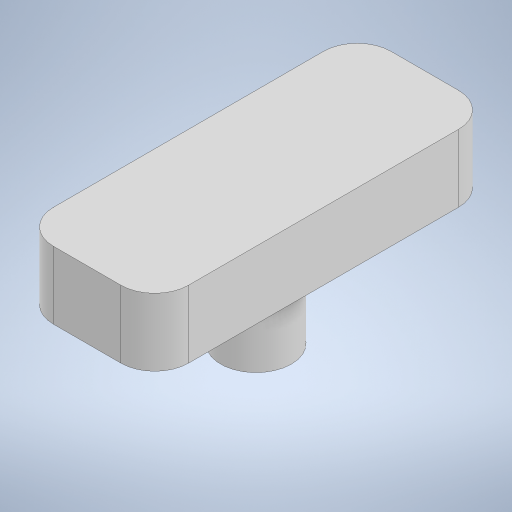
# Autodesk Inventor part: flipper_robot_v1_flipper_adapter
Saved by Autodesk Inventor 2023.1 (Build 271208000, 208)
## iProperties
Created: 2025-10-17
Part Number: flipper_robot_v1_flipper_adapter
Material: Generic
Document SubType Name: Modeling
Designer: Lars
Density: 1 g/cm^3
Appearance: Default
Author: Lars
Autodesk Inventor part; units mm, degrees
ref_plane "YZ Plane" through (0, 0, 0) normal (1, 0, 0) x (0, 1, 0)
ref_plane "XZ Plane" through (0, 0, 0) normal (0, 1, 0) x (-1, 0, 0)
ref_plane "XY Plane" through (0, 0, 0) normal (0, 0, 1) x (1, 0, 0)
sketch "Sketch1" plane through (0, 0, 0) normal (0, 1, 0) x (-1, 0, 0)
  line L0 (0.9994, -10) -> (3.0006, -10)
  ellipse E0 centre (2.9994, -8.9994) end of major axis (3.7074, -9.7074) minor radius 1 (3.0006, -10) -> (4, -9.0006) ccw
  line L1 (4, -9.0006) -> (4, -0.9994)
  ellipse E1 centre (2.9994, -1.0006) end of major axis (3.7074, -0.2926) minor radius 1 (4, -0.9994) -> (3.0006, 0) ccw
  line L2 (3.0006, 0) -> (0.9994, 0)
  ellipse E2 centre (1.0006, -1.0006) end of major axis (1.7086, -1.7086) minor radius 1 (0.9994, 0) -> (0, -0.9994) ccw
  line L3 (0, -0.9994) -> (0, -9.0006)
  ellipse E3 centre (1.0006, -8.9994) end of major axis (1.7086, -8.2914) minor radius 1 (0, -9.0006) -> (0.9994, -10) ccw
  circle A0 centre (2, -5) radius 1.75
  circle A1 centre (2, -5) radius 1.25
  line L4 (0, 0) -> (4, 0)
  line L5 (4, 0) -> (4, -10)
  line L6 (4, -10) -> (0, -10)
  line L7 (0, -10) -> (0, 0)
  circle A2 centre (2, -5) radius 1.05
  point P0 (0, -5)
  dimension "d3" = 1
  dimension "d7" = 1.0013
  dimension "d0" = 2.5
  dimension "d1" = 4
  dimension "d2" = 10
  dimension "d4" = 2
  dimension "d5" = 3.5
  dimension "d13" = 5
  dimension "d20" = 0.2
  constraints: 16 end point, 8 vertical, 7 horizontal, 3 centre point, 3 parallel, 2 coincident, 1 collinear, 1 midpoint, 1 perpendicular, 16 other
  measures "d0" diameter of A1
  measures "d1" distance between parallel lines of L1 L3
  measures "d2" distance between parallel lines of L0 L2
  measures "d4" distance of point (0, -5) A0.centre
  measures "d5" diameter of A0
  measures "d13" distance from line of A0.centre L6
  measures "d20" radial gap between concentric circles of A1 A2
extrude "Extrusion1" add sketch "Sketch1" along normal blind 2 contours E3 L3 E2 L2 E1 L1 E0 L0 | A0 | A1 | A2
extrude "Extrusion2" add sketch "Sketch1" against normal blind 2.5 contours A2
body "Solid1"
